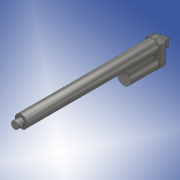
# Autodesk Inventor part: LinearActuator450
Saved by Autodesk Inventor 2017 SP1 (Build 210196100, 196)
## iProperties
Created: 2017-07-19
Part Number: LinearActuator450
Material: Steel, Carbon
Document SubType Name: Modeling
Designer: zallen
Density: 7.85 g/cm^3
Appearance: Semi-Polished
Catalog Web Link: http://www.eco-worthy.com/catalog/worthy-18450mm-stoke-linear-actuator-1500n-57mms-p-337.html
Vendor: ECO-WORTHY
Author: zallen
Autodesk Inventor part; units mm, degrees
ref_plane "YZ Plane" through (0, 0, 0) normal (1, 0, 0) x (0, 1, 0)
ref_plane "XZ Plane" through (0, 0, 0) normal (0, 1, 0) x (-1, 0, 0)
ref_plane "XY Plane" through (0, 0, 0) normal (0, 0, 1) x (1, 0, 0)
sketch "Sketch1" plane through (0, 0, 0) normal (0, 0, 1) x (1, 0, 0)
  line L0 (-10, -10) -> (10, -10)
  line L1 (10, -10) -> (10, 10)
  line L2 (10, 10) -> (-10, 10)
  line L3 (-10, 10) -> (-10, -10)
  line L4 (-10, -10) -> (10, 10) construction
  line L5 (10, -10) -> (-10, 10) construction
  line L6 (-20, 15) -> (-20, -32.5)
  line L7 (-20, 15) -> (-7.0096, 22.5)
  line L8 (-20, 15) -> (-5, 15) construction
  line L9 (-7.0096, 22.5) -> (7.0096, 22.5)
  line L10 (7.0096, 22.5) -> (20, 15)
  line L11 (20, 15) -> (20, -32.5)
  circle A0 centre (0, -32.5) radius 20 construction
  arc A1 (-20, -32.5) -> (20, -32.5) centre (0, -32.5) ccw
  point P0 (0, 0)
  point P1 (0, 22.5)
  point P2 (0, 10)
  dimension "d0" = 20
  dimension "d1" = 20
  dimension "d3" = 15
  dimension "d4" = 30
  dimension "d5" = 15
  dimension "d6" = 150
  dimension "d8" = 40
  dimension "d9" = 5
  dimension "d10" = 40
  dimension "d11" = 55
  constraints: 24 end point, 4 midpoint, 4 point on circle, 3 horizontal, 2 centre point, 2 parallel, 2 perpendicular, 1 concentric, 1 equal length, 1 tangent, 1 vertical, 1 vertical alignment
  measures "d0" distance of L2.end L1.end
  measures "d1" distance of L1.end L0.end
  measures "d3" distance of L6.start L7.end
  measures "d4" angle of L8 L7
  measures "d5" distance of L9.end L10.end
  measures "d6" angle of L9 L10
  measures "d8" distance between parallel lines of L11 L6
  measures "d9" vertical distance of L1.end L10.end
  measures "d10" diameter of A0
  measures "d11" distance of A1.centre point (0, 22.5)
extrude "Extrusion1" add sketch "Sketch1" along normal blind 18
sketch "Sketch2" plane through (0, 0, 18) normal (0, 0, 1) x (1, 0, 0)
  line L0 (-10, -10) -> (-10, 10) projected
  line L1 (-10, 10) -> (10, 10) projected
  line L2 (10, 10) -> (10, -10) projected
  line L3 (10, -10) -> (-10, -10) projected
  line L4 (-20, 15) -> (-20, -32.5) projected
  arc A0 (-20, -32.5) -> (20, -32.5) centre (0, -32.5) ccw projected
  line L5 (20, -32.5) -> (20, 15) projected
  line L6 (20, 15) -> (7.0096, 22.5) projected
  line L7 (7.0096, 22.5) -> (-7.0096, 22.5) projected
  line L8 (-7.0096, 22.5) -> (-20, 15) projected
  point P0 (0, 0)
extrude "Extrusion2" add sketch "Sketch2" against normal blind 36 contours L0 L1 L2 L3
sketch "Sketch3" plane through (10, -10, 0) normal (1, 0, 0) x (0, 0, -1)
  circle A0 centre (9, 10) radius 3.25
  line L0 (0, 20) -> (18, 20) projected
  line L1 (0, 0) -> (0, 20) projected
  point P0 (0, 10)
  point P1 (9, 20)
  point P2 (0, 10)
  dimension "d16" = 6.5
  constraints: 2 midpoint, 1 centre point, 1 horizontal alignment, 1 vertical alignment
  measures "d16" diameter of A0
extrude "Extrusion3" cut sketch "Sketch3" against normal through all
sketch "Sketch4" plane through (0, 0, 18) normal (0, 0, 1) x (1, 0, 0)
  circle A0 centre (0, 5) radius 17.5
  line L0 (7.0096, 22.5) -> (-7.0096, 22.5) projected
  point P0 (0, 0)
  point P1 (0, 22.5)
  dimension "d19" = 35
  constraints: 2 vertical alignment, 1 midpoint, 2 other
extrude "Extrusion4" add sketch "Sketch4" along normal blind 369
sketch "Sketch5" plane through (0, 0, 18) normal (0, 0, 1) x (1, 0, 0)
  circle A0 centre (0, -33) radius 19
  circle A1 centre (0, 5) radius 17.5 projected
  point P0 (0, 0)
  dimension "d22" = 38
  dimension "d23" = 38
  constraints: 1 centre point, 1 vertical alignment
  measures "d22" diameter of A0
  measures "d23" distance of A0.centre A1.centre
extrude "Extrusion5" add sketch "Sketch5" along normal blind 80 contours A0
sketch "Sketch6" plane through (0, 5, 387) normal (0, 0, 1) x (1, 0, 0)
  circle A0 centre (0, 0) radius 17.5 projected
  circle A1 centre (0, 0) radius 10
  point P0 (0, -5)
  dimension "d26" = 20
  constraints: 1 centre point, 1 coincident
  measures "d26" diameter of A1
extrude "Extrusion6" add sketch "Sketch6" along normal blind 18 contours A1
sketch "Sketch8" plane through (0, 0, 0) normal (1, 0, 0) x (0, 1, 0)
  line L0 (15, 405) -> (-5, 405) projected
  line L1 (-5, 387) -> (15, 387) projected
  circle A0 centre (5, 396) radius 3.25
  line L2 (15, 405) -> (15, 387)
  line L3 (15, 387) -> (15, 405) projected
  point P0 (0, 0)
  point P1 (15, 396)
  point P2 (5, 387)
  dimension "d29" = 6.5
  constraints: 2 end point, 2 midpoint, 1 centre point, 1 collinear, 1 horizontal alignment, 1 vertical alignment
  measures "d29" diameter of A0
extrude "Extrusion7" cut sketch "Sketch8" along normal through all both and the other way through all
body "Solid1"
